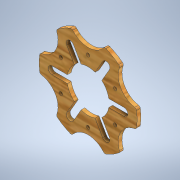
# Autodesk Inventor part: GenevaHolder
Saved by Autodesk Inventor 2020.1 (Build 241239000, 239)
## iProperties
Created: 2019-11-06
Part Number: GenevaHolder
Material: Plywood, Finish
Document SubType Name: Modeling
Designer: Paul Lefeuvre
Density: 0.552 g/cm^3
Appearance: Plywood - New
Author: Paul Lefeuvre
Autodesk Inventor part; units mm, degrees
ref_plane "YZ Plane" through (0, 0, 0) normal (1, 0, 0) x (0, 1, 0)
ref_plane "XZ Plane" through (0, 0, 0) normal (0, 1, 0) x (-1, 0, 0)
ref_plane "XY Plane" through (0, 0, 0) normal (0, 0, 1) x (1, 0, 0)
sketch "Sketch1" plane through (0, 0, 0) normal (0, 0, 1) x (1, 0, 0)
  circle A0 centre (0, 0) radius 175
  circle A1 centre (0, 136.9) radius 38.1
  line L0 (0, 0) -> (0, 152.9684) construction
  circle A2 centre (0, 0) radius 50
  line L1 (0, 0) -> (-42.671, 73.9083)
  line L2 (-31.9973, 38.421) -> (-50.0322, 69.6583)
  line L3 (-17.2749, 46.921) -> (-35.3098, 78.1583)
  arc A3 (-35.3098, 78.1583) -> (-50.0322, 69.6583) centre (-42.671, 73.9083) ccw
  line L4 (-16.7016, 47.1281) -> (-34.7901, 78.4583)
  arc A4 (-34.7901, 78.4583) -> (-50.5518, 69.3583) centre (-42.671, 73.9083) ccw
  line L5 (-50.5518, 69.3583) -> (-32.4633, 38.0281)
  line L6 (-49.1649, 9.1) -> (-85.342, 9.1)
  arc A5 (-85.342, 9.1) -> (-85.342, -9.1) centre (-85.342, 0) ccw
  line L7 (-85.342, -9.1) -> (-49.1649, -9.1)
  line L8 (-49.2722, 8.5) -> (-85.342, 8.5)
  arc A6 (-85.342, 8.5) -> (-85.342, -8.5) centre (-85.342, 0) ccw
  line L9 (-49.2722, -8.5) -> (-85.342, -8.5)
  line L10 (-32.4633, -38.0281) -> (-50.5518, -69.3583)
  arc A7 (-50.5518, -69.3583) -> (-34.7901, -78.4583) centre (-42.671, -73.9083) ccw
  line L11 (-34.7901, -78.4583) -> (-16.7016, -47.1281)
  line L12 (-31.9973, -38.421) -> (-50.0322, -69.6583)
  arc A8 (-50.0322, -69.6583) -> (-35.3098, -78.1583) centre (-42.671, -73.9083) ccw
  line L13 (-17.2749, -46.921) -> (-35.3098, -78.1583)
  line L14 (16.7016, -47.1281) -> (34.7901, -78.4583)
  arc A9 (34.7901, -78.4583) -> (50.5518, -69.3583) centre (42.671, -73.9083) ccw
  line L15 (50.5518, -69.3583) -> (32.4633, -38.0281)
  line L16 (17.2749, -46.921) -> (35.3098, -78.1583)
  arc A10 (35.3098, -78.1583) -> (50.0322, -69.6583) centre (42.671, -73.9083) ccw
  line L17 (31.9973, -38.421) -> (50.0322, -69.6583)
  line L18 (49.1649, -9.1) -> (85.342, -9.1)
  arc A11 (85.342, -9.1) -> (85.342, 9.1) centre (85.342, 0) ccw
  line L19 (85.342, 9.1) -> (49.1649, 9.1)
  line L20 (49.2722, -8.5) -> (85.342, -8.5)
  arc A12 (85.342, -8.5) -> (85.342, 8.5) centre (85.342, 0) ccw
  line L21 (49.2722, 8.5) -> (85.342, 8.5)
  line L22 (32.4633, 38.0281) -> (50.5518, 69.3583)
  arc A13 (50.5518, 69.3583) -> (34.7901, 78.4583) centre (42.671, 73.9083) ccw
  line L23 (34.7901, 78.4583) -> (16.7016, 47.1281)
  line L24 (31.9973, 38.421) -> (50.0322, 69.6583)
  arc A14 (50.0322, 69.6583) -> (35.3098, 78.1583) centre (42.671, 73.9083) ccw
  line L25 (17.2749, 46.921) -> (35.3098, 78.1583)
  arc A15 (49.2722, -8.5) -> (17.2749, 46.921) centre (49.2722, 28.4473) ccw construction
  circle A16 centre (0, 0) radius 93.842 construction
  arc A17 (17.2749, 46.921) -> (49.2722, -8.5) centre (49.2722, 28.4473) ccw construction
  circle A18 centre (49.2722, 28.4473) radius 19.9473 construction
  arc A19 (-26.9888, 110.0074) -> (26.9888, 110.0074) centre (0, 136.9) ccw
  circle A20 centre (0, 0) radius 74.4 construction
  circle A21 centre (0, 74.4) radius 3.9
  circle A22 centre (-64.4323, 37.2) radius 3.9
  circle A23 centre (-64.4323, -37.2) radius 3.9
  circle A24 centre (0, -74.4) radius 3.9
  circle A25 centre (64.4323, -37.2) radius 3.9
  circle A26 centre (64.4323, 37.2) radius 3.9
  circle A27 centre (0, 136.9) radius 47.2
  arc A28 (-36.4349, 106.8944) -> (-42.1081, 108.3798) centre (-40.2973, 103.7192) ccw
  arc A29 (42.1081, 108.3798) -> (36.4093, 106.863) centre (40.2973, 103.7192) ccw
  circle A30 centre (0, 136.9) radius 46.6 construction
  circle A31 centre (-118.5589, 68.45) radius 47.2
  arc A32 (-110.7908, 21.8936) -> (-114.9137, 17.7232) centre (-109.9722, 16.9611) ccw
  arc A33 (-72.8056, 90.6566) -> (-74.3414, 84.9629) centre (-69.6748, 86.7581) ccw
  circle A34 centre (-118.5589, -68.45) radius 47.2
  arc A35 (-74.3558, -85.0008) -> (-72.8056, -90.6566) centre (-69.6748, -86.7581) ccw
  arc A36 (-114.9137, -17.7232) -> (-110.7508, -21.9001) centre (-109.9722, -16.9611) ccw
  circle A37 centre (0, -136.9) radius 47.2
  arc A38 (36.4349, -106.8944) -> (42.1081, -108.3798) centre (40.2973, -103.7192) ccw
  arc A39 (-42.1081, -108.3798) -> (-36.4093, -106.863) centre (-40.2973, -103.7192) ccw
  circle A40 centre (118.5589, -68.45) radius 47.2
  arc A41 (110.7908, -21.8936) -> (114.9137, -17.7232) centre (109.9722, -16.9611) ccw
  arc A42 (72.8056, -90.6566) -> (74.3414, -84.9629) centre (69.6748, -86.7581) ccw
  circle A43 centre (118.5589, 68.45) radius 47.2
  arc A44 (74.3558, 85.0008) -> (72.8056, 90.6566) centre (69.6748, 86.7581) ccw
  arc A45 (114.9137, 17.7232) -> (110.7508, 21.9001) centre (109.9722, 16.9611) ccw
  arc A46 (-42.1081, 108.3798) -> (-72.8056, 90.6566) centre (0, 0) ccw
  arc A47 (-114.9137, 17.7232) -> (-114.9137, -17.7232) centre (0, 0) ccw
  arc A48 (-72.8056, -90.6566) -> (-42.1081, -108.3798) centre (0, 0) ccw
  arc A49 (42.1081, -108.3798) -> (72.8056, -90.6566) centre (0, 0) ccw
  arc A50 (114.9137, -17.7232) -> (114.9137, 17.7232) centre (0, 0) ccw
  arc A51 (72.8056, 90.6566) -> (42.1081, 108.3798) centre (0, 0) ccw
  point P0 (49.2722, -8.5)
  point P1 (31.9973, -38.421)
  point P2 (17.2749, -46.921)
  point P3 (-17.2749, -46.921)
  point P4 (-31.9973, -38.421)
  point P5 (-49.2722, -8.5)
  point P6 (17.2749, 46.921)
  point P7 (31.9973, 38.421)
  point P8 (49.2722, 8.5)
  point P9 (110.7946, 21.893)
  point P10 (74.3572, 85.0045)
  point P11 (36.4374, 106.8975)
  point P12 (-36.4374, 106.8975)
  point P13 (-74.3572, 85.0045)
  point P14 (-110.7946, 21.893)
  point P15 (-110.7946, -21.893)
  point P16 (-74.3572, -85.0045)
  point P17 (-36.4374, -106.8975)
  point P18 (36.4374, -106.8975)
  point P19 (74.3572, -85.0045)
  point P20 (110.7946, -21.893)
  dimension "d2" = 100
  dimension "d26" = 148.8
  dimension "d0" = 350
  dimension "d1" = 76.2
  dimension "d3" = 30
  dimension "d4" = 17
  dimension "d5" = 0.6
  dimension "d8" = 360
  dimension "d27" = 7.8
  dimension "d30" = 360
  dimension "d34" = 9.1
  dimension "d35" = 5
  dimension "d36" = 5
  dimension "d37" = 8.5
  dimension "d40" = 360
  constraints: 66 point on circle, 52 end point, 49 centre point, 10 tangent, 8 coincident, 3 parallel, 2 point on line, 1 vertical, 1 vertical alignment, 179 other
  measures "d0" diameter of A0
  measures "d1" diameter of A1
  measures "d3" angle of L0 L1
  measures "d4" distance between parallel lines of L2 L3
  measures "d5" distance between parallel lines of L3 L4
  measures "d27" diameter of A21
  measures "d34" radial gap between concentric circles of A1 A27
  measures "d35" radius of A28
  measures "d36" radius of A29
  measures "d37" radial gap between concentric circles of A30 A1
extrude "Extrusion1" add sketch "Sketch1" along normal blind 9 contours A45 A50 A41 A40 A42 A49 A38 A37 A39 A48 A35 A34 A36 A47 A32 A31 A33 A46 A28 A27 A29 A51 A44 A43
body "Solid1"
